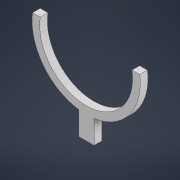
# Autodesk Inventor part: Clip_TestFitV1
Saved by Autodesk Inventor 2022 (Build 260153000, 153)
## iProperties
Created: 2023-05-05
Part Number: Clip_TestFitV1
Material: Generic
Document SubType Name: Modeling
Designer: User
Density: 1 g/cm^3
Appearance: Default
Author: User
Autodesk Inventor part; units mm, degrees
ref_plane "YZ Plane" through (0, 0, 0) normal (1, 0, 0) x (0, 1, 0)
ref_plane "XZ Plane" through (0, 0, 0) normal (0, 1, 0) x (-1, 0, 0)
ref_plane "XY Plane" through (0, 0, 0) normal (0, 0, 1) x (1, 0, 0)
sketch "Sketch1" plane through (0, 0, 0) normal (0, 0, 1) x (1, 0, 0)
  arc A0 (-30.1254, 4.7656) -> (30.1254, 4.7656) centre (0, 0) ccw
  line L0 (-30.1254, 4.7656) -> (-35.179, 4.7656)
  line L1 (30.1254, 4.7656) -> (35.2312, 4.8051)
  line L2 (30.1254, 4.7656) -> (35.2312, 4.8051) construction
  line L3 (5.2027, -35.5141) -> (5.2027, -50.5141)
  line L4 (5.2027, -50.5141) -> (-4.7973, -50.5141)
  line L5 (-4.7973, -50.5141) -> (-4.7973, -35.5141)
  line L6 (-4.7973, -35.5141) -> (-4.7973, -35.1747)
  line L7 (5.2027, -35.5141) -> (5.2027, -35.1747)
  arc A1 (-35.179, 4.7656) -> (-4.7973, -35.1747) centre (0, 0) ccw
  arc A2 (5.2027, -35.1747) -> (35.2312, 4.8051) centre (0, 0) ccw
  dimension "d0" = 61
  dimension "d5" = 10
  dimension "d6" = 15
  constraints: 16 end point, 6 point on circle, 3 centre point, 2 coincident, 1 parallel, 1 vertical
  measures "d0" diameter of A0
  measures "d5" distance of L3.end L4.end
  measures "d6" distance of L3.start L3.end
extrude "Extrusion1" add sketch "Sketch1" along normal blind 5
body "Solid1"
